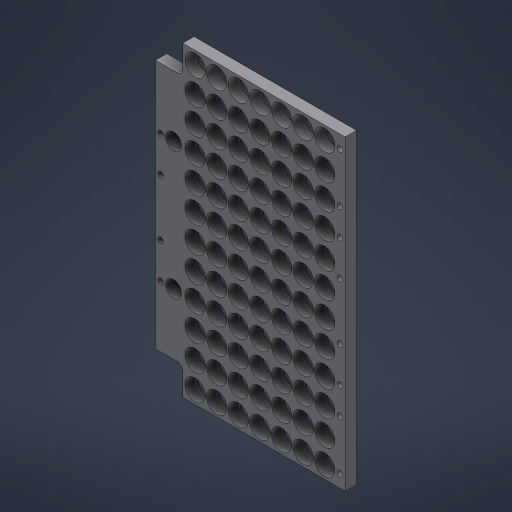
# Autodesk Inventor part: Platte1
Saved by Autodesk Inventor 2023.5 (Build 275446000, 446)
## iProperties
Created: 2025-03-19
Part Number: Platte1
Material: Generisch
Document SubType Name: Modeling
Designer: David Lill
Density: 1 g/cm^3
Appearance: Vorgabe
Author: David Lill
Autodesk Inventor part; units mm, degrees
ref_plane "YZ Plane" through (0, 0, 0) normal (1, 0, 0) x (0, 1, 0)
ref_plane "XZ Plane" through (0, 0, 0) normal (0, 1, 0) x (-1, 0, 0)
ref_plane "XY Plane" through (0, 0, 0) normal (0, 0, 1) x (1, 0, 0)
sketch "Skizze1" plane through (0, 0, 0) normal (0, 1, 0) x (-1, 0, 0)
  line L0 (167, 0) -> (0, 0)
  line L1 (0, 0) -> (0, -270)
  line L2 (0, -270) -> (167, -270)
  line L3 (167, -270) -> (167, 0)
  circle A0 centre (132, -11.25) radius 9
  circle A1 centre (132, -56.25) radius 9
  circle A2 centre (132, -101.25) radius 9
  circle A3 centre (132, -146.25) radius 9
  circle A4 centre (132, -191.25) radius 9
  circle A5 centre (132, -236.25) radius 9
  circle A6 centre (113, -11.25) radius 9
  circle A7 centre (113, -56.25) radius 9
  circle A8 centre (113, -101.25) radius 9
  circle A9 centre (113, -146.25) radius 9
  circle A10 centre (113, -191.25) radius 9
  circle A11 centre (113, -236.25) radius 9
  circle A12 centre (94, -11.25) radius 9
  circle A13 centre (94, -56.25) radius 9
  circle A14 centre (94, -101.25) radius 9
  circle A15 centre (94, -146.25) radius 9
  circle A16 centre (94, -191.25) radius 9
  circle A17 centre (94, -236.25) radius 9
  circle A18 centre (75, -11.25) radius 9
  circle A19 centre (75, -56.25) radius 9
  circle A20 centre (75, -101.25) radius 9
  circle A21 centre (75, -146.25) radius 9
  circle A22 centre (75, -191.25) radius 9
  circle A23 centre (75, -236.25) radius 9
  circle A24 centre (56, -11.25) radius 9
  circle A25 centre (56, -56.25) radius 9
  circle A26 centre (56, -101.25) radius 9
  circle A27 centre (56, -146.25) radius 9
  circle A28 centre (56, -191.25) radius 9
  circle A29 centre (56, -236.25) radius 9
  circle A30 centre (37, -11.25) radius 9
  circle A31 centre (37, -56.25) radius 9
  circle A32 centre (37, -101.25) radius 9
  circle A33 centre (37, -146.25) radius 9
  circle A34 centre (37, -191.25) radius 9
  circle A35 centre (37, -236.25) radius 9
  circle A36 centre (18, -11.25) radius 9
  circle A37 centre (18, -56.25) radius 9
  circle A38 centre (18, -101.25) radius 9
  circle A39 centre (18, -146.25) radius 9
  circle A40 centre (18, -191.25) radius 9
  circle A41 centre (18, -236.25) radius 9
  circle A42 centre (132, -33.75) radius 9
  circle A43 centre (113, -33.75) radius 9
  circle A44 centre (94, -33.75) radius 9
  circle A45 centre (75, -33.75) radius 9
  circle A46 centre (56, -33.75) radius 9
  circle A47 centre (37, -33.75) radius 9
  circle A48 centre (18, -33.75) radius 9
  circle A49 centre (132, -78.75) radius 9
  circle A50 centre (113, -78.75) radius 9
  circle A51 centre (94, -78.75) radius 9
  circle A52 centre (75, -78.75) radius 9
  circle A53 centre (56, -78.75) radius 9
  circle A54 centre (37, -78.75) radius 9
  circle A55 centre (18, -78.75) radius 9
  circle A56 centre (132, -123.75) radius 9
  circle A57 centre (113, -123.75) radius 9
  circle A58 centre (94, -123.75) radius 9
  circle A59 centre (75, -123.75) radius 9
  circle A60 centre (56, -123.75) radius 9
  circle A61 centre (37, -123.75) radius 9
  circle A62 centre (18, -123.75) radius 9
  circle A63 centre (132, -168.75) radius 9
  circle A64 centre (113, -168.75) radius 9
  circle A65 centre (94, -168.75) radius 9
  circle A66 centre (75, -168.75) radius 9
  circle A67 centre (56, -168.75) radius 9
  circle A68 centre (37, -168.75) radius 9
  circle A69 centre (18, -168.75) radius 9
  circle A70 centre (132, -213.75) radius 9
  circle A71 centre (113, -213.75) radius 9
  circle A72 centre (94, -213.75) radius 9
  circle A73 centre (75, -213.75) radius 9
  circle A74 centre (56, -213.75) radius 9
  circle A75 centre (37, -213.75) radius 9
  circle A76 centre (18, -213.75) radius 9
  circle A77 centre (132, -258.75) radius 9
  circle A78 centre (113, -258.75) radius 9
  circle A79 centre (94, -258.75) radius 9
  circle A80 centre (75, -258.75) radius 9
  circle A81 centre (56, -258.75) radius 9
  circle A82 centre (37, -258.75) radius 9
  circle A83 centre (18, -258.75) radius 9
  line L4 (-20, 0) -> (-187, 0)
  line L5 (-207, 0) -> (-374, 0)
  circle A84 centre (132, -11.25) radius 7.5
  point P0 (83.5, 0)
  dimension "d0" = 167
  dimension "d1" = 270
  dimension "d4" = 18
  dimension "d7" = 45
  dimension "d10" = 19
  dimension "d14" = 11.25
  dimension "d16" = 22.5
  dimension "d21" = 19
  dimension "d24" = 45
  dimension "d69" = 15
  dimension "d80" = 0
  dimension "d109" = 35
  constraints: 85 centre point, 14 coincident, 12 end point, 5 horizontal, 2 horizontal alignment, 2 parallel, 2 vertical, 1 equal radius, 1 midpoint, 1 perpendicular, 164 other
  measures "d0" distance of L0.start L0.end
  measures "d1" distance of L2.end L0.start
  measures "d4" diameter of A0
  measures "d7" distance of A0.centre A1.centre
  measures "d10" distance of A0.centre A6.centre
  measures "d14" distance from line of A0.centre L0
  measures "d16" distance of A42.centre A0.centre
  measures "d21" distance of A42.centre A43.centre
  measures "d24" distance of A42.centre A49.centre
  measures "d69" diameter of A84
  measures "d80" horizontal distance of A0.centre A42.centre
  measures "d109" distance from line of L3 A0.centre
extrude "Extrusion1" add sketch "Skizze1" along normal blind 10 contours L3 L2 L1 L0 | A0 | A1 | A2 | A3 | A4 | A5 | A6 | A7 | A8 | A9 | A10 | A11 | A12 | A13 | A14 | A15 | A16 | A17 | A18 | A19 | A20 | A21 | A22 | A23 | A24 | A25 | A26 | A27 | A28 | A29 | A30 | A31 | A32 | A33 | A34 | A35 | A36 | A37 | A38 | A39 | A40 | A41 | A42 | A43 | A44 | A45 | A46 | A47 | A48 | A49 | A50 | A51 | A52 | A53 | A54 | A55 | A56 | A57 | A58 | A59 | A60 | A61 | A62 | A63 | A64 | A65 | A66 | A67 | A68 | A69 | A70 | A71 | A72 | A73 | A74 | A75 | A76 | A77 | A78 | A79 | A80 | A81 | A82 | A83 | A84
hole "Bohrung1" at (-132, 0, -11.25) at (-132, 0, -33.75) at (-132, 0, -56.25) at (-132, 0, -78.75) at (-132, 0, -101.25) at (-132, 0, -123.75) at (-132, 0, -146.25) at (-132, 0, -168.75) at (-132, 0, -191.25) at (-132, 0, -213.75) at (-132, 0, -236.25) at (-132, 0, -258.75) direction (0, 1, 0) diameter 15 end through all counterbore diameter 18 counterbore depth 9
pattern_linear "Rechteckige Anordnung1" count 7 spacing 19 along (1, 0, 0) of "Bohrung1"
sketch "Skizze2" plane through (0, 10, 0) normal (0, 1, 0) x (1, 0, 0)
  circle A0 centre (-18, 236.25) radius 9 projected
  circle A1 centre (-18, 258.75) radius 9 projected
  circle A2 centre (-18, 213.75) radius 9 projected
  circle A3 centre (-18, 168.75) radius 9 projected
  circle A4 centre (-18, 123.75) radius 9 projected
  circle A5 centre (-18, 78.75) radius 9 projected
  circle A6 centre (-18, 33.75) radius 9 projected
  circle A7 centre (-18, 11.25) radius 9 projected
  circle A8 centre (-18, 56.25) radius 9 projected
  circle A9 centre (-18, 101.25) radius 9 projected
  circle A10 centre (-18, 146.25) radius 9 projected
  circle A11 centre (-18, 191.25) radius 9 projected
  circle A12 centre (-37, 236.25) radius 9 projected
  circle A13 centre (-37, 258.75) radius 9 projected
  circle A14 centre (-37, 213.75) radius 9 projected
  circle A15 centre (-37, 168.75) radius 9 projected
  circle A16 centre (-37, 123.75) radius 9 projected
  circle A17 centre (-37, 78.75) radius 9 projected
  circle A18 centre (-37, 33.75) radius 9 projected
  circle A19 centre (-37, 11.25) radius 9 projected
  circle A20 centre (-37, 56.25) radius 9 projected
  circle A21 centre (-37, 101.25) radius 9 projected
  circle A22 centre (-37, 146.25) radius 9 projected
  circle A23 centre (-37, 191.25) radius 9 projected
  circle A24 centre (-56, 236.25) radius 9 projected
  circle A25 centre (-56, 258.75) radius 9 projected
  circle A26 centre (-56, 213.75) radius 9 projected
  circle A27 centre (-56, 168.75) radius 9 projected
  circle A28 centre (-56, 123.75) radius 9 projected
  circle A29 centre (-56, 78.75) radius 9 projected
  circle A30 centre (-56, 33.75) radius 9 projected
  circle A31 centre (-56, 11.25) radius 9 projected
  circle A32 centre (-56, 56.25) radius 9 projected
  circle A33 centre (-56, 101.25) radius 9 projected
  circle A34 centre (-56, 146.25) radius 9 projected
  circle A35 centre (-56, 191.25) radius 9 projected
  circle A36 centre (-75, 236.25) radius 9 projected
  circle A37 centre (-75, 258.75) radius 9 projected
  circle A38 centre (-75, 213.75) radius 9 projected
  circle A39 centre (-75, 168.75) radius 9 projected
  circle A40 centre (-75, 123.75) radius 9 projected
  circle A41 centre (-75, 78.75) radius 9 projected
  circle A42 centre (-75, 33.75) radius 9 projected
  circle A43 centre (-75, 11.25) radius 9 projected
  circle A44 centre (-75, 56.25) radius 9 projected
  circle A45 centre (-75, 101.25) radius 9 projected
  circle A46 centre (-75, 146.25) radius 9 projected
  circle A47 centre (-75, 191.25) radius 9 projected
  circle A48 centre (-94, 236.25) radius 9 projected
  circle A49 centre (-94, 258.75) radius 9 projected
  circle A50 centre (-94, 213.75) radius 9 projected
  circle A51 centre (-94, 168.75) radius 9 projected
  circle A52 centre (-94, 123.75) radius 9 projected
  circle A53 centre (-94, 78.75) radius 9 projected
  circle A54 centre (-94, 33.75) radius 9 projected
  circle A55 centre (-94, 11.25) radius 9 projected
  circle A56 centre (-94, 56.25) radius 9 projected
  circle A57 centre (-94, 101.25) radius 9 projected
  circle A58 centre (-94, 146.25) radius 9 projected
  circle A59 centre (-94, 191.25) radius 9 projected
  circle A60 centre (-113, 236.25) radius 9 projected
  circle A61 centre (-113, 258.75) radius 9 projected
  circle A62 centre (-113, 213.75) radius 9 projected
  circle A63 centre (-113, 168.75) radius 9 projected
  circle A64 centre (-113, 123.75) radius 9 projected
  circle A65 centre (-113, 78.75) radius 9 projected
  circle A66 centre (-113, 33.75) radius 9 projected
  circle A67 centre (-113, 11.25) radius 9 projected
  circle A68 centre (-113, 56.25) radius 9 projected
  circle A69 centre (-113, 101.25) radius 9 projected
  circle A70 centre (-113, 146.25) radius 9 projected
  circle A71 centre (-113, 191.25) radius 9 projected
  circle A72 centre (-132, 236.25) radius 9 projected
  circle A73 centre (-132, 191.25) radius 9 projected
  circle A74 centre (-132, 146.25) radius 9 projected
  circle A75 centre (-132, 101.25) radius 9 projected
  circle A76 centre (-132, 56.25) radius 9 projected
  circle A77 centre (-132, 11.25) radius 9 projected
  circle A78 centre (-132, 33.75) radius 9 projected
  circle A79 centre (-132, 78.75) radius 9 projected
  circle A80 centre (-132, 123.75) radius 9 projected
  circle A81 centre (-132, 168.75) radius 9 projected
  circle A82 centre (-132, 213.75) radius 9 projected
  circle A83 centre (-132, 258.75) radius 9 projected
  line L0 (0, 0) -> (0, 270) projected
  line L1 (-167, 0) -> (0, 0) projected
  line L2 (-167, 270) -> (-167, 0) projected
  line L3 (0, 270) -> (-167, 270) projected
  line L4 (-144.5, 31.5) -> (-165.5, 31.5)
  line L5 (-165.5, 31.5) -> (-165.5, 58.5)
  line L6 (-165.5, 58.5) -> (-144.5, 58.5)
  line L7 (-144.5, 58.5) -> (-144.5, 31.5)
  line L8 (-167, 0) -> (0, 0) projected
  line L9 (-143, 0) -> (-143, 55)
  arc A84 (-143, 55) -> (-148, 60) centre (-148, 55) ccw
  line L10 (-148, 60) -> (-167, 60)
  line L11 (-167, 270) -> (-167, 0) projected
  line L12 (-167, 0) -> (0, 0) projected
  line L13 (0, 0) -> (0, 270) projected
  line L14 (-167, 270) -> (-167, 0) projected
  line L15 (0, 270) -> (-167, 270) projected
  line L16 (-167, 25) -> (-148, 25)
  arc A85 (-143, 20) -> (-148, 25) centre (-148, 20) ccw
  line L17 (0, 135) -> (-167, 135)
  line L18 (-144.5, 238.5) -> (-165.5, 238.5)
  line L19 (-165.5, 238.5) -> (-165.5, 211.5)
  line L20 (-165.5, 211.5) -> (-144.5, 211.5)
  line L21 (-144.5, 211.5) -> (-144.5, 238.5)
  line L22 (-143, 270) -> (-143, 215)
  arc A86 (-148, 210) -> (-143, 215) centre (-148, 215) ccw
  line L23 (-148, 210) -> (-167, 210)
  line L24 (-167, 245) -> (-148, 245)
  arc A87 (-148, 245) -> (-143, 250) centre (-148, 250) ccw
  arc A88 (-14.9586, 2.25) -> (-14.9586, 20.25) centre (-18, 11.25) ccw
  arc A89 (-14.9586, 2.25) -> (0, 11.25) centre (-14.9586, 19.1811) ccw
  arc A90 (0, 11.25) -> (-14.9586, 20.25) centre (-14.9586, 3.3189) ccw
  line L25 (-14.9586, 2.25) -> (-18, 2.25) construction
  circle A91 centre (-18, 11.25) radius 9 projected
  circle A92 centre (-4.65, 11.25) radius 2.5 construction
  arc A93 (-14.9586, 69.75) -> (-14.9586, 87.75) centre (-18, 78.75) ccw
  arc A94 (0, 78.75) -> (-14.9586, 87.75) centre (-14.9586, 70.8189) ccw
  arc A95 (-14.9586, 69.75) -> (0, 78.75) centre (-14.9586, 86.6811) ccw
  circle A96 centre (-4.65, 78.75) radius 2.5 construction
  arc A97 (-14.9586, 249.75) -> (-14.9586, 267.75) centre (-18, 258.75) ccw
  arc A98 (0, 258.75) -> (-14.9586, 267.75) centre (-14.9586, 250.8189) ccw
  arc A99 (-14.9586, 249.75) -> (0, 258.75) centre (-14.9586, 266.6811) ccw
  circle A100 centre (-4.65, 258.75) radius 2.5 construction
  arc A101 (-14.9586, 182.25) -> (-14.9586, 200.25) centre (-18, 191.25) ccw
  arc A102 (-14.9586, 182.25) -> (0, 191.25) centre (-14.9586, 199.1811) ccw
  arc A103 (0, 191.25) -> (-14.9586, 200.25) centre (-14.9586, 183.3189) ccw
  circle A104 centre (-4.65, 191.25) radius 2.5 construction
  line L26 (-135.0414, 87.75) -> (-158, 87.75)
  arc A105 (-158, 87.75) -> (-158, 69.75) centre (-158, 78.75) ccw
  line L27 (-158, 69.75) -> (-135.0414, 69.75)
  arc A106 (-135.0414, 87.75) -> (-135.0414, 69.75) centre (-132, 78.75) ccw
  line L28 (-135.0414, 182.25) -> (-158, 182.25)
  arc A107 (-158, 200.25) -> (-158, 182.25) centre (-158, 191.25) ccw
  line L29 (-158, 200.25) -> (-135.0414, 200.25)
  arc A108 (-135.0414, 200.25) -> (-135.0414, 182.25) centre (-132, 191.25) ccw
  circle A109 centre (-162.35, 78.75) radius 2.5 construction
  circle A110 centre (-162.35, 191.25) radius 2.5 construction
  circle A111 centre (-151, 78.75) radius 7
  circle A112 centre (-151, 191.25) radius 7
  line L30 (-83.5, 270) -> (-83.5, 0)
  line L31 (0, 219) -> (-4.65, 219)
  arc A113 (-4.65, 219) -> (-4.65, 211) centre (-4.65, 215) ccw
  line L32 (-4.65, 211) -> (0, 211)
  line L33 (0, 164) -> (-4.65, 164)
  arc A114 (-4.65, 164) -> (-4.65, 156) centre (-4.65, 160) ccw
  line L34 (-4.65, 156) -> (0, 156)
  line L35 (-167, 164) -> (-162.35, 164)
  arc A115 (-162.35, 156) -> (-162.35, 164) centre (-162.35, 160) ccw
  line L36 (-162.35, 156) -> (-167, 156)
  line L37 (0, 51) -> (-4.65, 51)
  arc A116 (-4.65, 59) -> (-4.65, 51) centre (-4.65, 55) ccw
  line L38 (-4.65, 59) -> (0, 59)
  line L39 (0, 106) -> (-4.65, 106)
  arc A117 (-4.65, 114) -> (-4.65, 106) centre (-4.65, 110) ccw
  line L40 (-4.65, 114) -> (0, 114)
  arc A118 (-162.35, 106) -> (-162.35, 114) centre (-162.35, 110) ccw
  line L41 (-167, 106) -> (-162.35, 106)
  line L42 (-162.35, 114) -> (-167, 114)
  point P0 (-167, 60)
  point P1 (-155, 31.5)
  point P2 (-165.5, 45)
  point P3 (-4.65, 258.75)
  point P4 (-8.5, 78.75)
  point P5 (-4.65, 215)
  point P6 (-4.65, 160)
  point P7 (-162.35, 55)
  point P8 (-162.35, 160)
  point P9 (-4.65, 55)
  point P10 (-4.65, 110)
  point P11 (0, 59)
  point P12 (0, 114)
  point P13 (0, 156)
  point P14 (0, 211)
  dimension "d81" = 21
  dimension "d82" = 27
  dimension "d83" = 24
  dimension "d84" = 5
  dimension "d85" = 60
  dimension "d92" = 12
  dimension "d93" = 45
  dimension "d101" = 25
  dimension "d110" = 9.5
  dimension "d112" = 5
  dimension "d114" = 78.85
  dimension "d118" = 157.7
  dimension "d119" = 14
  dimension "d121" = 16
  dimension "d124" = 55
  dimension "d125" = 55
  dimension "d126" = 4
  constraints: 66 end point, 58 symmetric about line, 53 point on circle, 34 centre point, 15 tangent, 11 coincident, 11 equal radius, 10 vertical alignment, 7 horizontal alignment, 6 midpoint, 5 perpendicular, 5 point on line, 4 horizontal, 3 concentric, 3 parallel, 2 vertical, 25 other
  measures "d81" distance of L5.end L6.end
  measures "d82" distance of L4.end L5.end
  measures "d83" distance between parallel lines of L2 L9
  measures "d84" radius of A84
  measures "d85" distance between parallel lines of L10 L8
  measures "d92" distance from line of L11 point (-155, 31.5)
  measures "d93" distance from line of point (-165.5, 45) L12
  measures "d101" distance between parallel lines of L8 L16
  measures "d110" radius of A88
  measures "d112" diameter of A92
  measures "d114" horizontal distance of L30.end point (-4.65, 11.25)
  measures "d118" horizontal distance of point (-4.65, 11.25) point (-162.35, 78.75)
  measures "d119" diameter of A111
  measures "d121" distance from line of L2 A111.centre
  measures "d124" distance from line of L15 point (-4.65, 215)
  measures "d125" distance of point (-4.65, 215) point (-4.65, 160)
  measures "d126" radius of A113
extrude "Extrusion2" cut sketch "Skizze2" against normal blind 10 contours L22 A87 L24 L2 L3 | L16 A85 L9 L1 L2 | A111 | A112
hole "Bohrung2" at (-4.65, 10, -11.25) at (-4.65, 10, -258.75) at (-162.35, 10, -78.75) at (-162.35, 10, -191.25) at (-4.65, 10, -191.25) at (-4.65, 10, -78.75) at (-4.65, 10, -215) at (-4.65, 10, -160) at (-4.65, 10, -110) at (-4.65, 10, -55) at (-162.35, 10, -160) at (-162.35, 10, -110) direction (0, -1, 0) diameter 5 end through all
equation "\"d7\" = 0.166667 * d1"
equation "\"d14\" = 0.5 * d16"
equation "\"d16\" = 0.5 * d7"
equation "\"d21\" = d10"
equation "\"d24\" = d7"
